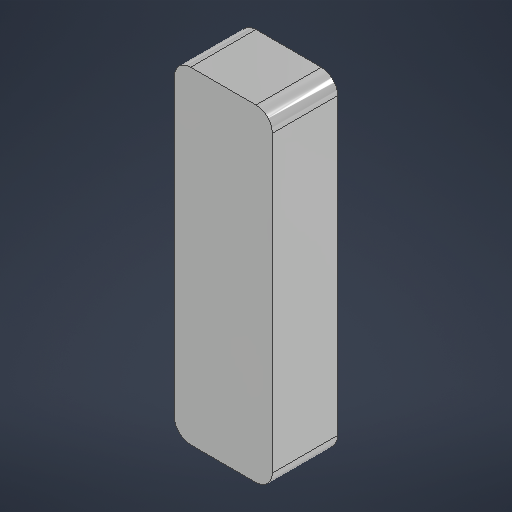
# Autodesk Inventor part: Magnet 10x3x2mm
Saved by Autodesk Inventor 2026.1 (Build 301233020, 233B)
## iProperties
Created: 2026-04-07
Part Number: Magnet 10x3x2mm
Material: Generic
Document SubType Name: Modeling
Designer: Bahaa
Mass: 0.0595708 g
Surface Area: 1.09854 cm^2
Volume: 0.0595708 cm^3
Density: 1 g/cm^3
Appearance: Default
Author: Bahaa
Autodesk Inventor part; units mm, degrees
ref_plane "YZ Plane" through (0, 0, 0) normal (1, 0, 0) x (0, 1, 0)
ref_plane "XZ Plane" through (0, 0, 0) normal (0, 1, 0) x (-1, 0, 0)
ref_plane "XY Plane" through (0, 0, 0) normal (0, 0, 1) x (1, 0, 0)
sketch "Sketch1" plane through (0, 0, 0) normal (0, 1, 0) x (-1, 0, 0)
  line L0 (1.5, 5) -> (-1.5, 5)
  line L1 (-1.5, 5) -> (-1.5, -5)
  line L2 (-1.5, -5) -> (1.5, -5)
  line L3 (1.5, -5) -> (1.5, 5)
  line L4 (1.5, 5) -> (-1.5, -5) construction
  line L5 (-1.5, 5) -> (1.5, -5) construction
  point P0 (0, 0)
  dimension "d0" = 3
  dimension "d1" = 10
  constraints: 12 end point, 2 midpoint, 2 parallel, 1 horizontal, 1 perpendicular
  measures "d0" distance of L2.end L1.end
  measures "d1" distance of L1.end L0.end
extrude "Extrusion1" add sketch "Sketch1" along normal blind 2
fillet "Fillet1" radius 0.5 4 edges at (1.5, 1, 5) (-1.5, 1, 5) (1.5, 1, -5) (-1.5, 1, -5)
body "Solid1"
